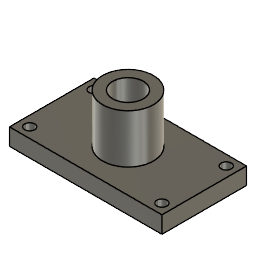
base camara (Autodesk Fusion 360 design; units mm, degrees)
Autodesk Fusion 360 part; units mm, degrees
note: some values were not read from the file. Set by a fixed rule: which face or edge a step refers to.
sketch "Boceto1" plane through (0, -44.5111, 133.5334) normal (0, -0.316228, 0.948683) x (1, 0, 0)
  line L0 (98.855, -216.4055) -> (90.855, -216.4055)
  line L1 (90.855, -216.4055) -> (90.855, -237.6861)
  line L2 (90.855, -237.6861) -> (179.145, -237.6861)
  line L3 (179.145, -237.6861) -> (179.145, -216.4055)
  line L4 (179.145, -216.4055) -> (171.145, -216.4055)
  line L5 (171.145, -216.4055) -> (98.855, -216.4055)
  line L6 (135, -216.4055) -> (135, -237.6861) construction
  line L7 (152.5, -237.0458) -> (117.5, -237.0458)
  line L8 (117.5, -237.0458) -> (117.5, -217.0458)
  line L9 (117.5, -217.0458) -> (152.5, -217.0458)
  line L10 (152.5, -217.0458) -> (152.5, -237.0458)
  line L11 (152.5, -237.0458) -> (117.5, -217.0458) construction
  line L12 (117.5, -237.0458) -> (152.5, -217.0458) construction
  circle A0 centre (121.5, -220.5458) radius 1.5
  line L13 (117.5, -227.0458) -> (152.5, -227.0458) construction
  circle A1 centre (148.5, -220.5458) radius 1.5
  circle A2 centre (121.5, -233.5458) radius 1.5
  circle A3 centre (148.5, -233.5458) radius 1.5
  point P0 (135, -227.0458)
  dimension "d1" = 20
  dimension "d2" = 35
  dimension "d5" = 3
  dimension "d8" = 3.5
  dimension "d9" = 4
  constraint midpoint L5 L6.start
  constraint midpoint L2 L6.end
  constraint horizontal L7
  constraint perpendicular L7 L8
  constraint parallel L7 L9
  constraint parallel L8 L10
  constraint coincident L11 P0
  constraint coincident L12 P0
  constraint midpoint L6 P0
  constraint midpoint L8 L13.start
  constraint midpoint L10 L13.end
  constraint symmetric L6 A0 A1
  constraint symmetric A0 L13 A2
  constraint symmetric L13 A1 A3
  measures "d1" distance of L7 L9
  measures "d2" distance of L8 L10
  measures "d5" diameter of A0
  measures "d8" distance of L9 A0.centre
  measures "d9" distance of L8 A0.centre
sketch "Boceto2" plane through (0, -46.0923, 138.2768) normal (0, -0.316228, 0.948683) x (1, 0, 0)
  circle A0 centre (121.5, -233.5458) radius 1.5
  circle A1 centre (148.5, -233.5458) radius 1.5
  circle A2 centre (148.5, -220.5458) radius 1.5
  circle A3 centre (121.5, -220.5458) radius 1.5
  line L0 (152.5, -217.0458) -> (117.5, -217.0458)
  line L1 (117.5, -217.0458) -> (117.5, -237.0458)
  line L2 (117.5, -237.0458) -> (152.5, -237.0458)
  line L3 (152.5, -237.0458) -> (152.5, -217.0458)
  circle A4 centre (121.5, -220.5458) radius 3
  line L4 (135, -217.0458) -> (135, -237.0458) construction
  line L5 (117.5, -227.0458) -> (152.5, -227.0458) construction
  circle A5 centre (148.5, -220.5458) radius 3
  circle A6 centre (121.5, -233.5458) radius 3
  circle A7 centre (148.5, -233.5458) radius 3
  circle A8 centre (135, -227.0458) radius 7.5
  circle A9 centre (135, -227.0458) radius 4.5
  dimension "d12" = 1.5
  dimension "d15" = 15
  dimension "d16" = -3
  constraint midpoint L0 L4.start
  constraint midpoint L2 L4.end
  constraint midpoint L1 L5.start
  constraint midpoint L3 L5.end
  constraint symmetric A4 L4 A5
  constraint symmetric A4 L5 A6
  constraint symmetric L5 A5 A7
  constraint midpoint L5 A8.centre
  measures "d12" distance of A3
  measures "d15" diameter of A8
sketch "Boceto3" plane through (0, 0, 70.1) normal (0, 0, 1) x (-1, 0, 0)
  line L0 (-99.155, 234.8114) -> (-179.145, 234.8114)
  line L1 (-179.145, 234.8114) -> (-179.145, 30)
  line L2 (-179.145, 30) -> (-99.155, 30)
  line L3 (-99.155, 30) -> (-99.155, 77.19)
  line L4 (-99.155, 77.19) -> (-109.155, 77.19)
  line L5 (-109.155, 77.19) -> (-109.155, 192.81)
  line L6 (-109.155, 192.81) -> (-99.155, 192.81)
  line L7 (-99.155, 192.81) -> (-99.155, 234.8114)
  circle A0 centre (-174.995, 55.245) radius 2.75
  circle A1 centre (-175.145, 219.21) radius 2.75
  ellipse E0 centre (-148.5, 255.3204) end of major axis (-151.5, 255.3204) minor radius 2.846
  ellipse E1 centre (-121.5, 267.6533) end of major axis (-124.5, 267.6533) minor radius 2.846
  ellipse E2 centre (-121.5, 255.3204) end of major axis (-124.5, 255.3204) minor radius 2.846
  ellipse E3 centre (-148.5, 267.6533) end of major axis (-151.5, 267.6533) minor radius 2.846
  line L8 (-152.5, 252) -> (-117.5, 252)
  line L9 (-117.5, 252) -> (-117.5, 270.9737)
  line L10 (-117.5, 270.9737) -> (-152.5, 270.9737)
  line L11 (-152.5, 270.9737) -> (-152.5, 252)
  line L12 (-135, 252) -> (-135, 270.9737)
  line L13 (-117.5, 261.4868) -> (-152.5, 261.4868)
  circle A2 centre (-135, 261.4868) radius 4.5
  circle A3 centre (-135, 261.4868) radius 7.5
  dimension "d21" = 9
  dimension "d22" = 3
  constraint midpoint L12 A2.centre
  measures "d21" diameter of A2
extrude "Extruir7" add sketch "Boceto3" along normal blind 8 contours L12 L13 A2 A3 | L12 L13 A2 A3 | L12 L13 A2 A3 | L12 L13 A2 A3 makes body 1
extrude "Extruir8" add 1 faces at (141.4746, -261.131, 70.1) along direction (0, 0, -1) blind 11.39 on bodies 1 bodies 1
sketch "Boceto4" plane through (0, 0, 58.71) normal (0, 0, -1) x (1, 0, 0)
  circle A0 centre (135, 261.4868) radius 4.5
  circle A1 centre (135, 261.4868) radius 7.5
  line L0 (112.5, 273.9868) -> (157.5, 273.9868)
  line L1 (157.5, 273.9868) -> (157.5, 248.9868)
  line L2 (157.5, 248.9868) -> (112.5, 248.9868)
  line L3 (112.5, 248.9868) -> (112.5, 273.9868)
  line L4 (112.5, 273.9868) -> (157.5, 248.9868) construction
  line L5 (148, 256.4868) -> (122, 256.4868)
  line L6 (122, 256.4868) -> (122, 266.4868)
  line L7 (122, 266.4868) -> (148, 266.4868)
  line L8 (148, 266.4868) -> (148, 256.4868)
  line L9 (148, 256.4868) -> (122, 266.4868) construction
  line L10 (122, 256.4868) -> (148, 266.4868) construction
  circle A2 centre (135, 261.4868) radius 4.5
  point P0 (135, 261.4868)
  point P1 (135, 261.4868)
  dimension "d32" = 45
  dimension "d33" = 25
  dimension "d34" = 26
  dimension "d35" = 10
  constraint horizontal L0
  constraint perpendicular L0 L1
  constraint parallel L0 L2
  constraint parallel L1 L3
  constraint coincident L4 P1
  constraint coincident P0 A0.centre
  constraint horizontal L5
  constraint perpendicular L5 L6
  constraint parallel L5 L7
  constraint parallel L6 L8
  constraint coincident L9 P1
  constraint coincident L10 P1
  constraint coincident P1 P0
  measures "d32" distance of L1.end L2.end
  measures "d33" distance of L0.end L1.end
  measures "d34" distance of L6.end L7.end
  measures "d35" distance of L5.end L6.end
extrude "Extruir9" add sketch "Boceto4" against normal blind 5 bodies 1
extrude "Extruir10" add sketch "Boceto4" along normal blind -5 and the other way blind 3 contours A1 L5 L7 L8 | A1 L5 L6 L7 bodies 1
sketch "Boceto5" plane through (0, 0, 63.71) normal (0, 0, 1) x (-1, 0, 0)
  circle A0 centre (-135, 261.4868) radius 7.5
  line L0 (-157.5, 248.9868) -> (-112.5, 248.9868)
  line L1 (-112.5, 248.9868) -> (-112.5, 273.9868)
  line L2 (-112.5, 273.9868) -> (-157.5, 273.9868)
  line L3 (-157.5, 273.9868) -> (-157.5, 248.9868)
  line L4 (-157.5, 273.9868) -> (-154.5, 273.9868)
  line L5 (-154.5, 273.9868) -> (-154.5, 270.9868)
  circle A1 centre (-154.5, 270.9868) radius 1.5
  line L6 (-157.5, 261.4868) -> (-156.5179, 261.4868)
  line L7 (-156.5179, 261.4868) -> (-112.5, 261.4868)
  line L8 (-135, 248.9868) -> (-135, 273.9868)
  circle A2 centre (-115.5, 270.9868) radius 1.5
  circle A3 centre (-115.5, 251.9868) radius 1.5
  circle A4 centre (-154.5, 251.9868) radius 1.5
  dimension "d42" = 3
  dimension "d43" = 3
  dimension "d44" = 3
  dimension "d45" = 3
  dimension "d46" = 3
  dimension "d47" = 3
  constraint coincident L2.end L3.start
  constraint perpendicular L3 L4
  constraint perpendicular L4 L5
  constraint coincident L5.end A1.centre
  constraint midpoint L3 L6.start
  constraint perpendicular L3 L6
  constraint midpoint L1 L7.end
  constraint midpoint L0 L8.start
  constraint midpoint L2 L8.end
  constraint symmetric A1 L7 A4
  constraint symmetric A1 L8 A2
  constraint symmetric L7 A2 A3
  measures "d42" distance of L2.end L4.end
  measures "d43" distance of L4.end L5.end
  measures "d44" diameter of A1
  measures "d45" diameter of A2
  measures "d46" diameter of A3
  measures "d47" diameter of A4
extrude "Extruir11" cut sketch "Boceto5" against normal blind 10 contours A1 | A2 | A3 | A4 bodies 1
sketch "Boceto6" plane through (0, 0, 0) normal (0, 0, 1) x (1, 0, 0)
  line L0 (150, -200) -> (150, -186.5)
  line L1 (150, -186.5) -> (145, -186.5)
  line L2 (145, -186.5) -> (145, -200)
  line L3 (145, -200) -> (150, -200)
  dimension "d50" = 13.5
  dimension "d51" = 5
  constraint vertical L0
  constraint perpendicular L0 L1
  constraint perpendicular L1 L2
  constraint perpendicular L0 L3
  measures "d50" distance of L0.start L0.end
  measures "d51" distance of L0.end L1.end
sketch "Boceto7" plane through (0, 0, 0) normal (0, 0, -1) x (1, 0, 0)
  line L0 (150, 200) -> (145, 200)
  line L1 (145, 200) -> (145, 186.5)
  line L2 (145, 186.5) -> (150, 186.5)
  line L3 (150, 186.5) -> (150, 200)
  line L4 (150, 186.5) -> (145, 186.5)
  line L5 (145, 186.5) -> (145, 188.5)
  line L6 (145, 188.5) -> (150, 188.5)
  line L7 (150, 188.5) -> (150, 186.5)
  dimension "d54" = 2
  constraint horizontal L4
  constraint vertical L5
  constraint horizontal L6
  constraint vertical L7
  constraint coincident L2.end L3.start
  measures "d54" distance of L2.end L6.end
sketch "Boceto8" plane through (0, -188.5, 0) normal (0, -1, 0) x (1, 0, 0)
  line L0 (145, -5) -> (145, -6)
  line L1 (145, -6) -> (150, -6)
  line L2 (150, -6) -> (150, -5)
  line L3 (150, -6) -> (145, -6)
  line L4 (145, -6) -> (145, -4)
  line L5 (145, -4) -> (150, -4)
  line L6 (150, -4) -> (150, -6)
  line L7 (150, -5) -> (145, -5)
  dimension "d59" = 2
  constraint horizontal L3
  constraint vertical L4
  constraint horizontal L5
  constraint vertical L6
  constraint coincident L1.end L2.start
  measures "d59" distance of L1.end L5.end
move_body "Desplazar1" bodies 1 to x (1, 0, 0) y (0, 1, 0) z (0, 0, 1) at (0, 0, -50)
sketch "Boceto9" plane through (0, -247, 0) normal (0, -1, 0) x (1, 0, 0)
  line L0 (119, 8.7) -> (124, 8.7)
  line L1 (124, 8.7) -> (124, 13.7)
  line L2 (124, 13.7) -> (119, 13.7)
  line L3 (119, 13.7) -> (119, 8.7)
  line L4 (122.75, 12.45) -> (120.25, 12.45)
  line L5 (120.25, 12.45) -> (120.25, 9.95)
  line L6 (120.25, 9.95) -> (122.75, 9.95)
  line L7 (122.75, 9.95) -> (122.75, 12.45)
  line L8 (122.75, 12.45) -> (120.25, 9.95) construction
  line L9 (120.25, 12.45) -> (122.75, 9.95) construction
  point P0 (121.5, 11.2)
  dimension "d62" = 2.5
  dimension "d63" = 2.5
  constraint horizontal L4
  constraint perpendicular L4 L5
  constraint parallel L4 L6
  constraint parallel L5 L7
  constraint coincident L8 P0
  constraint coincident L9 P0
  measures "d62" distance of L5.end L6.end
  measures "d63" distance of L4.end L5.end
extrude "Extruir16" cut sketch "Boceto9" along normal blind 7 contours L4 L5 L6 L7 bodies 1
extrude "Extruir17" add sketch "Boceto9" along normal blind 5 contours L4 L5 L6 L7 makes body 2
sketch "Boceto10" plane through (0, -247, 0) normal (0, -1, 0) x (1, 0, 0)
  line L0 (146, 8.7) -> (151, 8.7)
  line L1 (151, 8.7) -> (151, 13.7)
  line L2 (151, 13.7) -> (146, 13.7)
  line L3 (146, 13.7) -> (146, 8.7)
  line L4 (147.25, 9.95) -> (149.75, 9.95)
  line L5 (149.75, 9.95) -> (149.75, 12.45)
  line L6 (149.75, 12.45) -> (147.25, 12.45)
  line L7 (147.25, 12.45) -> (147.25, 9.95)
  line L8 (147.25, 9.95) -> (149.75, 12.45) construction
  line L9 (149.75, 9.95) -> (147.25, 12.45) construction
  point P0 (148.5, 11.2)
  dimension "d68" = 2.5
  dimension "d69" = 2.5
  constraint horizontal L4
  constraint perpendicular L4 L5
  constraint parallel L4 L6
  constraint parallel L5 L7
  constraint coincident L8 P0
  constraint coincident L9 P0
  measures "d68" distance of L5.end L6.end
  measures "d69" distance of L4.end L5.end
extrude "Extruir18" cut sketch "Boceto10" along normal blind 7 contours L4 L5 L6 L7 bodies 1
extrude "Extruir19" add sketch "Boceto10" along normal blind 5 contours L4 L5 L6 L7 makes body 3
move_body "Desplazar6" bodies 3 to x (1, 0, 0) y (0, 1, 0) z (0, 0, 1) at (0, -2, 0)
move_body "Desplazar7" bodies 2 to x (1, 0, 0) y (0, 1, 0) z (0, 0, 1) at (0, -2, 0)
sketch "Boceto11" plane through (0, 0, 8.71) normal (0, 0, -1) x (1, 0, 0)
  circle A0 centre (154.5, 251.9868) radius 1.5
  circle A1 centre (115.5, 270.9868) radius 1.5
  circle A2 centre (154.5, 270.9868) radius 1.5
  circle A3 centre (115.5, 251.9868) radius 1.5
  arc A4 (140.5902, 256.4868) -> (140.5902, 266.4868) centre (135, 261.4868) ccw
  line L0 (140.5902, 266.4868) -> (148, 266.4868)
  line L1 (148, 266.4868) -> (148, 256.4868)
  line L2 (148, 256.4868) -> (140.5902, 256.4868)
  line L3 (112.5, 248.9868) -> (157.5, 248.9868)
  line L4 (157.5, 248.9868) -> (157.5, 273.9868)
  line L5 (157.5, 273.9868) -> (112.5, 273.9868)
  line L6 (112.5, 273.9868) -> (112.5, 248.9868)
  line L7 (129.4098, 256.4868) -> (122, 256.4868)
  line L8 (122, 256.4868) -> (122, 266.4868)
  line L9 (122, 266.4868) -> (129.4098, 266.4868)
  arc A5 (129.4098, 266.4868) -> (129.4098, 256.4868) centre (135, 261.4868) ccw
  line L10 (153, 254) -> (117, 254)
  line L11 (117, 254) -> (117, 268.9737)
  line L12 (117, 268.9737) -> (153, 268.9737)
  line L13 (153, 268.9737) -> (153, 254)
  line L14 (153, 254) -> (117, 268.9737) construction
  line L15 (117, 254) -> (153, 268.9737) construction
  point P0 (135, 261.4868)
  constraint horizontal L10
  constraint perpendicular L10 L11
  constraint parallel L10 L12
  constraint parallel L11 L13
  constraint coincident L14 P0
  constraint coincident L15 P0
  constraint coincident P0 A4.centre
extrude "Extruir20" cut sketch "Boceto11" against normal blind 3 contours A4 L0 L1 L2 | L7 L8 L9 A5 | L10 L11 L12 L13 bodies 1
extrude "Extruir21" add 3 faces at (133.3592, -262.8648, 11.71) (123.8333, -261.4868, 11.71) (146.1667, -261.4868, 11.71) along direction (0, 0, -1) blind 3 on bodies 1 bodies 1
extrude "Extruir22" add 4 faces at (148.9167, -254, 11.1233) (148.0833, -254, 12.2033) (121.9167, -254, 11.1233) (121.9167, -254, 11.9567) along direction (0, 1, 0) blind 5.013 on bodies 1 bodies 1
combine "Combinar1" operation add target body 1 tool bodies 2 3
